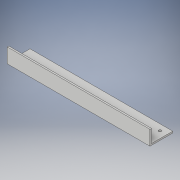
# Autodesk Inventor part: angle iron with  holes 1
Saved by Autodesk Inventor 2018 (Build 220112000, 112)
## iProperties
Created: 2019-02-23
Part Number: angle iron with  holes 1
Material: Generic
Document SubType Name: Modeling
Designer: s-2513225
Density: 1 g/cm^3
Appearance: Default
Author: s-2513225
Autodesk Inventor part; units mm, degrees
ref_plane "YZ Plane" through (0, 0, 0) normal (1, 0, 0) x (0, 1, 0)
ref_plane "XZ Plane" through (0, 0, 0) normal (0, 1, 0) x (-1, 0, 0)
ref_plane "XY Plane" through (0, 0, 0) normal (0, 0, 1) x (1, 0, 0)
sketch "Sketch1" plane through (0, 0, 0) normal (0, 1, 0) x (-1, 0, 0)
  line L0 (0, 0) -> (279.4, 0)
  line L1 (279.4, 0) -> (279.4, -44.577)
  line L2 (279.4, -44.577) -> (0, -44.577)
  line L3 (0, -44.577) -> (0, 0)
  dimension "d0" = 279.4
  dimension "d1" = 44.577
  constraints: 8 end point, 2 parallel, 1 horizontal, 1 perpendicular
  measures "d0" distance of L1.end L2.end
  measures "d1" distance of L0.end L1.end
extrude "Extrusion1" add sketch "Sketch1" along normal blind 3.175
sketch "Sketch2" plane through (0, 3.175, 0) normal (0, 1, 0) x (1, 0, 0)
  line L0 (-279.4, 0) -> (0, 0) projected
  line L1 (-279.4, 0) -> (0, 0)
  line L2 (0, 0) -> (0, 3.175)
  line L3 (0, 3.175) -> (-279.4, 3.175)
  line L4 (-279.4, 3.175) -> (-279.4, 0)
  dimension "d4" = 279.4
  dimension "d5" = 3.175
  constraints: 8 end point, 2 parallel, 1 horizontal, 1 perpendicular
  measures "d4" distance of L3.end L2.end
  measures "d5" distance of L2.end L1.end
extrude "Extrusion2" add sketch "Sketch2" along normal blind 25.4
sketch "Sketch3" plane through (0, 3.175, 0) normal (0, 1, 0) x (1, 0, 0)
  line L0 (0, 44.577) -> (-279.4, 44.577) construction
  line L1 (0, 44.577) -> (-13.081, 44.577) construction
  line L2 (-13.081, 44.577) -> (-13.081, 32.5755) construction
  line L3 (0, 3.175) -> (0, 44.577) construction
  line L4 (0, 44.577) -> (-24.003, 44.577) construction
  line L5 (-24.003, 44.577) -> (-24.003, 20.574) construction
  circle A0 centre (-24.003, 20.574) radius 2.5797
  circle A1 centre (-13.081, 32.5755) radius 2.5797
  point P0 (0, 0)
  dimension "d10" = 13.081
  dimension "d11" = 24.003
  dimension "d12" = 5.1594
  dimension "d13" = 5.1594
  constraints: 8 end point, 2 centre point, 2 coincident, 2 perpendicular, 2 point on line
  measures "d10" distance of L0.start L1.end
  measures "d11" distance of L0.start L4.end
  measures "d12" diameter of A0
  measures "d13" diameter of A1
extrude "Extrusion3" cut sketch "Sketch3" against normal blind 25.4
body "Solid1"
